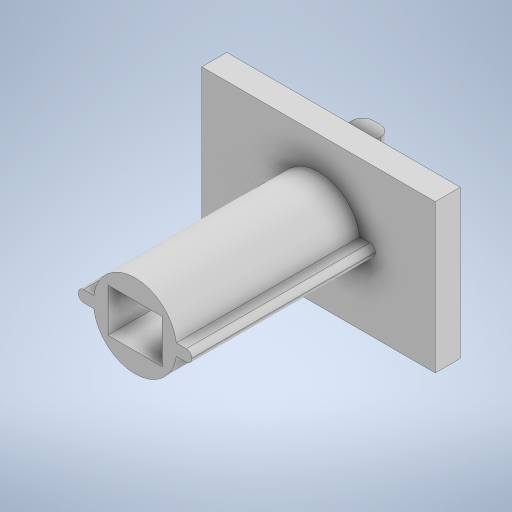
# Autodesk Inventor part: power_switch
Saved by Autodesk Inventor 2024 (Build 280153000, 153)
## iProperties
Created: 2023-06-19
Part Number: power_switch
Material: Generic
Document SubType Name: Modeling
Designer: jconvertino
Density: 1 g/cm^3
Appearance: Default
Author: jconvertino
Autodesk Inventor part; units mm, degrees
ref_plane "YZ Plane" through (0, 0, 0) normal (1, 0, 0) x (0, 1, 0)
ref_plane "XZ Plane" through (0, 0, 0) normal (0, 1, 0) x (-1, 0, 0)
ref_plane "XY Plane" through (0, 0, 0) normal (0, 0, 1) x (1, 0, 0)
sketch "Sketch1" plane through (0, 0, 0) normal (0, 0, 1) x (1, 0, 0)
  line L0 (-21.2139, 7.4194) -> (14.3461, 7.4194)
  line L1 (14.3461, 7.4194) -> (14.3461, -15.1866)
  line L2 (14.3461, -15.1866) -> (-21.2139, -15.1866)
  line L3 (-21.2139, -15.1866) -> (-21.2139, 7.4194)
  point P0 (0, 0)
  dimension "d0" = 22.606
  dimension "d1" = 35.56
  constraints: 8 end point, 2 parallel, 1 horizontal, 1 perpendicular
  measures "d0" distance of L0.end L1.end
  measures "d1" distance of L0.start L0.end
extrude "Extrusion1" add sketch "Sketch1" along normal blind 3.81
sketch "Sketch2" plane through (0, 0, 3.81) normal (0, 0, 1) x (1, 0, 0)
  line L0 (14.3461, 7.4194) -> (-21.2139, 7.4194) projected
  line L1 (-21.2139, -15.1866) -> (14.3461, -15.1866) projected
  line L2 (14.3461, -15.1866) -> (14.3461, 7.4194) projected
  line L3 (-21.2139, 7.4194) -> (-21.2139, -15.1866) projected
  line L4 (5.2021, -2.9946) -> (5.2021, -4.7726)
  line L5 (-12.0699, -4.7726) -> (-12.0699, -2.9946)
  line L6 (5.2021, -4.7726) -> (2.8536, -4.7726)
  line L7 (-9.7213, -4.7726) -> (-12.0699, -4.7726)
  line L8 (-12.0699, -2.9946) -> (-9.7213, -2.9946)
  line L9 (2.8536, -2.9946) -> (5.2021, -2.9946)
  arc A0 (-9.7213, -4.7726) -> (2.8536, -4.7726) centre (-3.4339, -3.8836) ccw
  arc A1 (2.8536, -2.9946) -> (-9.7213, -2.9946) centre (-3.4339, -3.8836) ccw
  point P0 (0, 0)
  dimension "d5" = 11.303
  dimension "d6" = 11.303
  dimension "d7" = 17.78
  dimension "d8" = 17.78
  dimension "d9" = 17.272
  dimension "d10" = 1.778
  dimension "d13" = 9.144
  dimension "d14" = 9.144
  constraints: 12 end point, 5 parallel, 4 point on circle, 2 centre point, 2 horizontal, 2 perpendicular
  measures "d5" distance from line of L0 A0.centre
  measures "d6" distance from line of L1 A0.centre
  measures "d7" distance from line of L2 A0.centre
  measures "d8" distance from line of L3 A0.centre
  measures "d9" distance between parallel lines of L4 L5
  measures "d10" distance of L4.start L4.end
  measures "d13" distance between parallel lines of L2 L4
  measures "d14" distance between parallel lines of L3 L5
extrude "Extrusion2" add sketch "Sketch2" along normal blind 27.94 contours L4 L6 A0 L7 L5 L8 A1 L9
sketch "Sketch3" plane through (0, 0, 31.75) normal (0, 0, 1) x (1, 0, 0)
  line L0 (-7.5614, -0.5816) -> (0.6936, -0.5816)
  line L1 (0.6936, -0.5816) -> (0.6936, -7.1856)
  line L2 (0.6936, -7.1856) -> (-7.5614, -7.1856)
  line L3 (-7.5614, -7.1856) -> (-7.5614, -0.5816)
  line L4 (-12.0699, -2.9946) -> (-12.0699, -4.7726) projected
  line L5 (5.2021, -4.7726) -> (5.2021, -2.9946) projected
  arc A0 (2.8536, -2.9946) -> (-9.7213, -2.9946) centre (-3.4339, -3.8836) ccw projected
  arc A1 (-9.7213, -4.7726) -> (2.8536, -4.7726) centre (-3.4339, -3.8836) ccw projected
  point P0 (0, 0)
  point P1 (-12.0699, -3.8836)
  point P2 (5.2021, -3.8836)
  point P3 (-3.4339, 2.4664)
  point P4 (-3.4339, -10.2336)
  dimension "d17" = 8.255
  dimension "d18" = 6.604
  dimension "d19" = 4.5085
  dimension "d20" = 4.5085
  dimension "d21" = 3.048
  dimension "d22" = 3.048
  constraints: 8 end point, 2 midpoint, 2 parallel, 2 point on circle, 1 horizontal, 1 perpendicular
  measures "d17" distance of L0.start L0.end
  measures "d18" distance of L0.end L1.end
  measures "d19" distance from line of point (-12.07, -3.884) L3
  measures "d20" distance from line of point (5.202, -3.884) L1
  measures "d21" distance from line of L0 point (-3.434, 2.466)
  measures "d22" distance from line of point (-3.434, -10.234) L2
extrude "Extrusion3" cut sketch "Sketch3" against normal blind 27.94
sketch "Sketch4" plane through (0, 0, 0) normal (0, 0, -1) x (-1, 0, 0)
  line L0 (1.2749, 4.4984) -> (5.5929, 4.4984)
  line L1 (5.5929, 4.4984) -> (5.5929, -12.2656)
  line L2 (5.5929, -12.2656) -> (1.2749, -12.2656)
  line L3 (1.2749, -12.2656) -> (1.2749, 4.4984)
  line L4 (-14.3461, 7.4194) -> (21.2139, 7.4194) projected
  line L5 (21.2139, -15.1866) -> (-14.3461, -15.1866) projected
  line L6 (21.2139, 7.4194) -> (21.2139, -15.1866) projected
  line L7 (-14.3461, -15.1866) -> (-14.3461, 7.4194) projected
  point P0 (0, 0)
  point P1 (21.2139, -3.8836)
  dimension "d25" = 4.318
  dimension "d26" = 16.764
  dimension "d27" = 2.921
  dimension "d28" = 2.921
  dimension "d29" = 15.621
  dimension "d30" = 15.621
  constraints: 8 end point, 2 parallel, 1 horizontal, 1 midpoint, 1 perpendicular
  measures "d25" distance of L0.start L0.end
  measures "d26" distance of L0.end L1.end
  measures "d27" distance between parallel lines of L4 L0
  measures "d28" distance between parallel lines of L5 L2
  measures "d29" distance from line of point (21.214, -3.884) L1
  measures "d30" distance between parallel lines of L7 L3
extrude "Extrusion4" add sketch "Sketch4" along normal blind 5.08 contours L0 L1 L2 L3
fillet "Fillet1" radius 1.5875 2 edges at (-5.5929, -3.8836, -5.08) (-1.2749, -3.8836, -5.08)
fillet "Fillet2" radius 0.8255 4 edges at (-12.0699, -4.7726, 17.78) (-12.0699, -2.9946, 17.78) (5.2021, -4.7726, 17.78) (5.2021, -2.9946, 17.78)
sketch "Sketch5" plane through (0, 0, 0) normal (0, 0, -1) x (-1, 0, 0)
  line L0 (6.4184, -8.3286) -> (6.4184, 0.5614)
  line L1 (6.4184, 0.5614) -> (9.5934, -3.8836)
  line L2 (9.5934, -3.8836) -> (6.4184, -8.3286)
  line L3 (0.4494, -8.3286) -> (0.4494, 0.5614)
  line L4 (0.4494, 0.5614) -> (-2.7256, -3.8836)
  line L5 (-2.7256, -3.8836) -> (0.4494, -8.3286)
  line L6 (5.5929, -12.2656) -> (5.5929, 4.4984) projected
  line L7 (1.2749, 4.4984) -> (1.2749, -12.2656) projected
  line L8 (21.2139, -15.1866) -> (-14.3461, -15.1866) projected
  line L9 (-14.3461, 7.4194) -> (21.2139, 7.4194) projected
  point P0 (0, 0)
  dimension "d35" = 3.175
  dimension "d36" = 8.89
  dimension "d37" = 0.8255
  dimension "d38" = 0.8255
  dimension "d39" = 6.858
  dimension "d40" = 6.858
  dimension "d41" = 6.858
  dimension "d42" = 6.858
  dimension "d43" = 4.445
  dimension "d44" = 4.445
  dimension "d45" = 4.445
  constraints: 12 end point, 2 parallel, 2 vertical
  measures "d35" distance from line of L3 L4.end
  measures "d36" distance of L3.start L3.end
  measures "d37" distance between parallel lines of L6 L0
  measures "d38" distance between parallel lines of L7 L3
  measures "d39" distance from line of L8 L0.start
  measures "d40" distance from line of L9 L0.end
  measures "d41" distance from line of L8 L3.start
  measures "d42" distance from line of L9 L3.end
  measures "d43" vertical distance of L1.end L0.start
  measures "d44" vertical distance of L0.end L1.end
  measures "d45" vertical distance of L4.end L3.start
extrude "Extrusion5" add sketch "Sketch5" along normal blind 0.635
body "Solid1"
